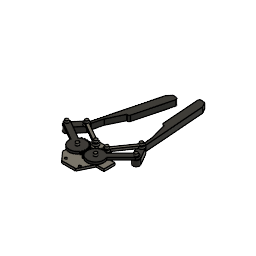
Record 11 (Autodesk Fusion 360 design; units mm, degrees)
part number: 2025-10-11-10-03-09-255
part number: 2025-10-12-12-27-50-455
part number: 2025-10-12-12-41-17-092
part number: 2025-10-12-12-45-11-913
part number: 2025-10-12-13-17-20-818
part number: 2025-10-12-13-49-26-949
Autodesk Fusion 360 part; units mm, degrees
sketch "Sketch2" plane through (0, 0, 0) normal (0, 1, 0) x (1, 0, 0)
  line L0 (0, 0) -> (14.2, 0)
  line L1 (14.2, 0) -> (14.2, 20)
  line L2 (0, 0) -> (-12.1733, -24.993)
  line L3 (-12.1733, -24.993) -> (-37.1733, -24.993)
  line L4 (-37.1733, -24.993) -> (-51.09, -9.7775)
  line L5 (-51.09, -9.7775) -> (-51.09, 20.2225)
  line L6 (-51.09, 20.2225) -> (-31.8645, 38.417)
  line L7 (-31.8645, 38.417) -> (-11.8645, 38.417)
  line L8 (-11.8645, 38.417) -> (7.148, 20)
  line L9 (7.148, 20) -> (14.2, 20)
  dimension "d11" = 14.2
  dimension "d12" = 20
  dimension "d13" = 27.8
  dimension "d14" = 25
  dimension "d15" = 20.62
  dimension "d16" = 30
  dimension "d17" = 26.47
  dimension "d18" = 20
  dimension "d20" = 26.47
  dimension "d21" = 63.41
  dimension "d22" = 65.29
  constraint coincident L0.start L2.start
  constraint horizontal L0
  constraint perpendicular L0 L1
  constraint perpendicular L1 L3
  constraint vertical L5
  constraint horizontal L7
  constraint perpendicular L1 L9
  measures "d11" distance of L0.start L0.end
  measures "d12" distance of L0.end L1.end
  measures "d13" distance of L0.start L2.end
  measures "d14" distance of L2.end L3.end
  measures "d15" distance of L3.end L4.end
  measures "d16" distance of L4.end L5.end
  measures "d17" distance of L5.end L6.end
  measures "d18" distance of L6.end L7.end
  measures "d20" distance of L7.end L8.end
  measures "d21" distance of L3 L7
  measures "d22" distance of L1 L5
extrude "Extrude1" add sketch "Sketch2" along normal blind 4 makes body 1
sketch "Sketch3" plane through (0, 4, 0) normal (0, 1, 0) x (-1, 0, 0)
  line L0 (0, 0) -> (-14.2, 0)
  line L1 (-14.2, 0) -> (-14.2, -20)
  line L2 (-14.2, -20) -> (-7.148, -20)
  line L3 (-7.148, -20) -> (11.8645, -38.417)
  line L4 (11.8645, -38.417) -> (31.8645, -38.417)
  line L5 (31.8645, -38.417) -> (51.09, -20.2225)
  line L6 (51.09, -20.2225) -> (51.09, 9.7775)
  line L7 (51.09, 9.7775) -> (37.1733, 24.993)
  line L8 (37.1733, 24.993) -> (12.1733, 24.993)
  line L9 (12.1733, 24.993) -> (0, 0)
  circle A0 centre (31.8645, -31.417) radius 3
  circle A1 centre (11.8645, -31.417) radius 3
  circle A2 centre (44, -10.2225) radius 3
  line L10 (15, -7) -> (0, -7)
  arc A3 (0, -7) -> (0, -13) centre (0, -10) ccw
  line L11 (0, -13) -> (15, -13)
  arc A4 (15, -13) -> (15, -7) centre (15, -10) ccw
  line L12 (15, -10) -> (0, -10) construction
  circle A5 centre (37.1733, 17.3853) radius 2
  circle A6 centre (12.1733, 17.3853) radius 2
  dimension "d25" = 6
  dimension "d26" = 6
  dimension "d27" = 7
  dimension "d28" = 7
  dimension "d29" = 6
  dimension "d30" = 10
  dimension "d31" = 7.09
  dimension "d32" = 6
  dimension "d33" = 14.2
  dimension "d34" = 10
  dimension "d35" = 4
  dimension "d36" = 4
  constraint tangent L10 A3
  constraint tangent A3 L11
  constraint parallel L10 L11
  constraint tangent L11 A4
  constraint tangent L10 A4
  constraint horizontal L12
  measures "d25" diameter of A0
  measures "d26" diameter of A1
  measures "d27" distance of L4.end A0.centre
  measures "d28" distance of L3.end A1.centre
  measures "d29" diameter of A2
  measures "d30" vertical distance of L5.end A2.centre
  measures "d31" distance of L6 A2.centre
  measures "d32" diameter of A3
  measures "d33" distance of L1 A3.centre
  measures "d34" distance of L2 A3.centre
  measures "d35" diameter of A5
  measures "d36" diameter of A6
extrude "Extrude2" cut sketch "Sketch3" against normal blind 33 contours A0 | A1 | A2 | L10 A3 L11 A4 | A5 | A6 bodies 1
sketch "Sketch1" plane through (0, 0, 0) normal (0, 1, 0) x (1, 0, 0) in component "part2"
  circle A0 centre (20.4961, 19.7492) radius 3
  line L0 (20.4961, 19.7492) -> (20.4961, -25.2508)
  circle A1 centre (20.4961, -25.2508) radius 3
  line L1 (17.9959, 15.4192) -> (17.9959, -20.9208)
  line L2 (22.9963, 15.4192) -> (22.9963, -20.9208)
  arc A2 (22.9963, 15.4192) -> (17.9959, 15.4192) centre (20.4961, 19.7492) ccw
  arc A3 (17.9959, -20.9208) -> (22.9963, -20.9208) centre (20.4961, -25.2508) ccw
  dimension "d39" = 10
  dimension "d40" = 6
  dimension "d41" = 45
  dimension "d42" = 10
  dimension "d43" = 6
  dimension "d44" = 36.34
  constraint concentric A0 A2
  constraint coincident A0.centre L0.start
  constraint vertical L0
  constraint coincident L0.end A1.centre
  constraint concentric A1 A3
  constraint vertical L1
  constraint symmetric L0 L1.start L2.start
  constraint symmetric L0 L1.end L2.end
  measures "d39" diameter of A2
  measures "d40" diameter of A0
  measures "d41" distance of A0.centre L0.end
  measures "d42" diameter of A3
  measures "d43" diameter of A1
  measures "d44" distance of L1.start L1.end
extrude "Extrude1'" add sketch "Sketch1" along normal blind 4 separate body makes body 2 in component "part2"
sketch "Sketch1 (2)" plane through (0, 0, 0) normal (0, 1, 0) x (1, 0, 0) in component "part 3"
  circle A0 centre (32, 23) radius 3
  dimension "d47" = 6
  measures "d47" diameter of A0
extrude "Extrude1''" add sketch "Sketch1 (2)" along normal blind 18 separate body makes body 3 in component "part 3"
sketch "Sketch1 (3)" plane through (0, 0, 0) normal (0, 1, 0) x (1, 0, 0) in component "part 4"
  circle A0 centre (-75.4732, 20.9598) radius 3
  line L0 (-75.4732, 20.9598) -> (-75.4732, -31.0102)
  circle A1 centre (-75.4732, -31.0102) radius 3
  line L1 (-80.3495, -29.9048) -> (-80.3495, 6.7746)
  line L2 (-70.597, -29.9048) -> (-70.597, 6.7746)
  arc A2 (-80.3495, -29.9048) -> (-70.597, -29.9048) centre (-75.4732, -31.0102) ccw
  line L3 (-75.4732, 20.9598) -> (-75.4732, 40)
  line L4 (-76.5054, 35.9243) -> (-76.5054, 37.4643)
  line L5 (-76.5054, 37.4643) -> (-76.5054, 35.9243)
  line L6 (-76.5054, 37.4643) -> (-75.9732, 37.9343)
  line L7 (-75.9732, 37.9343) -> (-75.4732, 37.9343)
  line L8 (-74.4411, 37.4643) -> (-74.4411, 35.9243)
  line L9 (-74.4411, 37.4643) -> (-74.9732, 37.9343)
  line L10 (-74.9732, 37.9343) -> (-75.4732, 37.9343)
  line L11 (-80.2193, 35.1892) -> (-80.6049, 36.6801)
  line L12 (-80.6049, 36.6801) -> (-80.2074, 37.2684)
  line L13 (-80.2074, 37.2684) -> (-79.7233, 37.3936)
  line L14 (-79.2392, 37.5188) -> (-79.7233, 37.3936)
  line L15 (-78.6063, 37.197) -> (-79.2392, 37.5188)
  line L16 (-78.6063, 37.197) -> (-78.2208, 35.706)
  line L17 (-83.6309, 33.5476) -> (-84.3775, 34.8945)
  line L18 (-84.3775, 34.8945) -> (-84.1399, 35.5636)
  line L19 (-84.1399, 35.5636) -> (-83.7026, 35.806)
  line L20 (-83.2653, 36.0484) -> (-83.7026, 35.806)
  line L21 (-82.572, 35.8953) -> (-83.2653, 36.0484)
  line L22 (-82.572, 35.8953) -> (-81.8254, 34.5484)
  line L23 (-86.5228, 31.1042) -> (-87.5829, 32.2212)
  line L24 (-87.5829, 32.2212) -> (-87.5204, 32.9285)
  line L25 (-87.5204, 32.9285) -> (-87.1577, 33.2726)
  line L26 (-86.795, 33.6168) -> (-87.1577, 33.2726)
  line L27 (-86.0854, 33.6422) -> (-86.795, 33.6168)
  line L28 (-86.0854, 33.6422) -> (-85.0254, 32.5251)
  line L29 (-88.7108, 28.0144) -> (-90.0168, 28.8305)
  line L30 (-90.0168, 28.8305) -> (-90.1333, 29.5309)
  line L31 (-90.1333, 29.5309) -> (-89.8684, 29.9549)
  line L32 (-89.6034, 30.3789) -> (-89.8684, 29.9549)
  line L33 (-88.9228, 30.5812) -> (-89.6034, 30.3789)
  line L34 (-88.9228, 30.5812) -> (-87.6168, 29.7651)
  line L35 (-90.0555, 24.4753) -> (-91.5242, 24.9384)
  line L36 (-91.5242, 24.9384) -> (-91.8124, 25.5873)
  line L37 (-91.8124, 25.5873) -> (-91.6621, 26.0641)
  line L38 (-91.5117, 26.541) -> (-91.6621, 26.0641)
  line L39 (-90.9034, 26.9072) -> (-91.5117, 26.541)
  line L40 (-90.9034, 26.9072) -> (-89.4347, 26.4441)
  line L41 (-90.4712, 20.7122) -> (-92.0091, 20.7928)
  line L42 (-92.0091, 20.7928) -> (-92.4506, 21.3489)
  line L43 (-92.4506, 21.3489) -> (-92.4244, 21.8482)
  line L44 (-92.3983, 22.3475) -> (-92.4244, 21.8482)
  line L45 (-91.901, 22.8543) -> (-92.3983, 22.3475)
  line L46 (-91.901, 22.8543) -> (-90.3632, 22.7738)
  line L47 (-89.9315, 16.9649) -> (-91.4406, 16.6579)
  line L48 (-91.4406, 16.6579) -> (-92.0072, 17.0857)
  line L49 (-92.0072, 17.0857) -> (-92.1069, 17.5757)
  line L50 (-92.2066, 18.0656) -> (-92.1069, 17.5757)
  line L51 (-91.8521, 18.6808) -> (-92.2066, 18.0656)
  line L52 (-91.8521, 18.6808) -> (-90.3431, 18.9878)
  line L53 (-88.4707, 13.4721) -> (-89.8549, 12.797)
  line L54 (-89.8549, 12.797) -> (-90.5106, 13.0693)
  line L55 (-90.5106, 13.0693) -> (-90.7298, 13.5187)
  line L56 (-90.949, 13.9681) -> (-90.7298, 13.5187)
  line L57 (-90.7598, 14.6525) -> (-90.949, 13.9681)
  line L58 (-90.7598, 14.6525) -> (-89.3757, 15.3275)
  line L59 (-86.182, 10.4563) -> (-87.353, 9.4562)
  line L60 (-87.353, 9.4562) -> (-88.056, 9.5556)
  line L61 (-88.056, 9.5556) -> (-88.3807, 9.9358)
  line L62 (-88.7054, 10.316) -> (-88.3807, 9.9358)
  line L63 (-88.6937, 11.0259) -> (-88.7054, 10.316)
  line L64 (-88.6937, 11.0259) -> (-87.5226, 12.0261)
  line L65 (-83.211, 8.1096) -> (-84.0943, 6.8481)
  line L66 (-84.0943, 6.8481) -> (-84.7998, 6.7684)
  line L67 (-84.7998, 6.7684) -> (-85.2094, 7.0552)
  line L68 (-85.619, 7.342) -> (-85.2094, 7.0552)
  line L69 (-85.7853, 8.0322) -> (-85.619, 7.342)
  line L70 (-85.7853, 8.0322) -> (-84.902, 9.2937)
  arc A3 (-70.597, 6.7746) -> (-74.4411, 35.9243) centre (-75.4732, 20.9598) ccw
  arc A4 (-76.5054, 35.9243) -> (-78.2208, 35.706) centre (-75.4732, 20.9598) ccw
  arc A5 (-80.2193, 35.1892) -> (-81.8254, 34.5484) centre (-75.4732, 20.9598) ccw
  arc A6 (-83.6309, 33.5476) -> (-85.0254, 32.5251) centre (-75.4732, 20.9598) ccw
  arc A7 (-86.5228, 31.1042) -> (-87.6168, 29.7651) centre (-75.4732, 20.9598) ccw
  arc A8 (-88.7108, 28.0144) -> (-89.4347, 26.4441) centre (-75.4732, 20.9598) ccw
  arc A9 (-90.0555, 24.4753) -> (-90.3632, 22.7738) centre (-75.4732, 20.9598) ccw
  arc A10 (-90.4712, 20.7122) -> (-90.3431, 18.9878) centre (-75.4732, 20.9598) ccw
  arc A11 (-89.9315, 16.9649) -> (-89.3757, 15.3275) centre (-75.4732, 20.9598) ccw
  arc A12 (-88.4707, 13.4721) -> (-87.5226, 12.0261) centre (-75.4732, 20.9598) ccw
  arc A13 (-86.182, 10.4563) -> (-84.902, 9.2937) centre (-75.4732, 20.9598) ccw
  arc A14 (-83.211, 8.1096) -> (-80.3495, 6.7746) centre (-75.4732, 20.9598) ccw
  dimension "d50" = 30
  dimension "d51" = 6
  dimension "d52" = 10
  dimension "d53" = 6
  dimension "d54" = 51.97
  dimension "d55" = 1.54
  dimension "d56" = 0.47
  dimension "d57" = 0.5
  dimension "d58" = 0.71
  dimension "d60" = 145
  constraint concentric A0 A3
  constraint coincident A0.centre L0.start
  constraint vertical L0
  constraint coincident L0.end A1.centre
  constraint concentric A1 A2
  constraint parallel L0 L1
  constraint symmetric L0 L1.start L2.start
  constraint symmetric L0 L1.end L2.end
  constraint parallel L0 L3
  constraint vertical L4
  constraint coincident L4.start A3
  constraint coincident L3 L7.end
  constraint perpendicular L3 L7
  constraint symmetric L3 L4.start L8.end
  constraint symmetric L3 L4.end L8.start
  constraint symmetric L3 L6.end L9.end
  constraint symmetric L3 L7.end L10.end
  constraint concentric A3 A4
  constraint concentric A4 A5
  constraint concentric A5 A6
  constraint concentric A6 A7
  constraint concentric A7 A8
  constraint concentric A8 A9
  constraint concentric A9 A10
  constraint concentric A10 A11
  constraint concentric A11 A12
  constraint concentric A12 A13
  constraint concentric A13 A14
  measures "d50" diameter of A3
  measures "d51" diameter of A0
  measures "d52" diameter of A2
  measures "d53" diameter of A1
  measures "d54" distance of A0.centre L0.end
  measures "d55" distance of L4.start L4.end
  measures "d56" vertical distance of L4.end L6.end
  measures "d57" distance of L6.end L7.end
  measures "d58" distance of L4.end L6.end
extrude "Extrude1'''" add sketch "Sketch1 (3)" along normal blind 4 separate body makes body 4 in component "part 4"
sketch "Sketch1 (4)" plane through (0, 0, 0) normal (0, 1, 0) x (1, 0, 0) in component "part 5"
  line L0 (79.2313, -48.7678) -> (79.2313, -23.7678)
  arc A0 (79.2313, -23.7678) -> (67.2313, -23.7678) centre (73.2313, -23.7678) ccw
  line L1 (67.2313, -23.7678) -> (67.2313, -48.7678)
  arc A1 (67.2313, -48.7678) -> (79.2313, -48.7678) centre (73.2313, -48.7678) ccw
  line L2 (73.2313, -48.7678) -> (73.2313, -23.7678) construction
  line L3 (69.067, -19.4483) -> (20.2413, 82.4588)
  line L4 (20.2413, 82.4588) -> (20.2413, 92.3588)
  line L5 (26.0982, 96.1925) -> (20.2413, 92.3588)
  line L6 (30.4467, 94.9786) -> (59.6439, 34.0394)
  arc A2 (30.4467, 94.9786) -> (26.0982, 96.1925) centre (27.7412, 93.6824) ccw
  line L7 (77.8305, -27.1163) -> (64.8679, -0.0613)
  line L8 (58.2346, 30.0376) -> (57.3328, 29.6055)
  line L9 (57.3328, 29.6055) -> (64.8679, -0.0613)
  arc A3 (58.2346, 30.0376) -> (59.6439, 34.0394) centre (56.9384, 32.7431) ccw
  point P0 (28.9658, 98.0695)
  point P1 (60.9401, 31.3339)
  dimension "d63" = 25
  dimension "d64" = 12
  dimension "d65" = 113
  dimension "d66" = 154.4
  dimension "d67" = 58.99
  dimension "d68" = 9.9
  dimension "d69" = 74
  dimension "d70" = 3
  dimension "d71" = 7
  dimension "d72" = 30
  dimension "d73" = 4.59
  dimension "d74" = 3
  dimension "d75" = 1
  constraint tangent L0 A0
  constraint tangent A0 L1
  constraint parallel L0 L1
  constraint tangent L1 A1
  constraint tangent L0 A1
  constraint vertical L2
  constraint coincident A0 L3.start
  constraint vertical L4
  constraint parallel L3 L6
  constraint coincident P0 L5
  constraint coincident P0 L6
  constraint tangent L5 A2
  constraint tangent L6 A2
  constraint parallel L3 L7
  constraint perpendicular L6 L8
  constraint coincident P1 L6
  constraint coincident P1 L8
  constraint tangent L6 A3
  constraint tangent L8 A3
  measures "d63" distance of A1.centre A0.centre
  measures "d64" diameter of A0
  measures "d65" distance of L3.start L3.end
  measures "d66" angle of L1 L3
  measures "d67" distance of L0 L3.end
  measures "d68" distance of L3.end L4.end
  measures "d69" distance of P0 P1
  measures "d70" radius of A2
  measures "d71" distance of L4.end L5.start
  measures "d72" distance of L7.start L7.end
  measures "d73" distance of L3 L7
  measures "d74" radius of A3
  measures "d75" distance of L8.end L8.start
extrude "Extrude1''''" add sketch "Sketch1 (4)" along normal blind 10 separate body makes body 5 in component "part 5"
sketch "Sketch2 (2)" plane through (0, 10, 0) normal (0, 1, 0) x (-1, 0, 0) in component "part 5"
  line L0 (-57.3328, -29.6055) -> (-58.2346, -30.0376)
  arc A0 (-58.2346, -30.0376) -> (-59.6439, -34.0394) centre (-56.9384, -32.7431) ccw
  line L1 (-59.6439, -34.0394) -> (-30.4467, -94.9786)
  arc A1 (-30.4467, -94.9786) -> (-26.0982, -96.1925) centre (-27.7412, -93.6824) ccw
  line L2 (-26.0982, -96.1925) -> (-20.2413, -92.3588)
  line L3 (-20.2413, -92.3588) -> (-20.2413, -82.4588)
  line L4 (-20.2413, -82.4588) -> (-69.067, 19.4483)
  arc A2 (-69.067, 19.4483) -> (-67.2313, 23.7678) centre (-73.2313, 23.7678) ccw
  line L5 (-67.2313, 23.7678) -> (-67.2313, 48.7678)
  arc A3 (-67.2313, 48.7678) -> (-79.2313, 48.7678) centre (-73.2313, 48.7678) ccw
  line L6 (-79.2313, 48.7678) -> (-79.2313, 23.7678)
  arc A4 (-79.2313, 23.7678) -> (-73.3521, 17.7691) centre (-73.2313, 23.7678) ccw
  line L7 (-73.3521, 17.7691) -> (-64.8679, 0.0613)
  line L8 (-64.8679, 0.0613) -> (-57.3328, -29.6055)
  circle A5 centre (-73.2313, 48.7678) radius 3
  circle A6 centre (-73.2313, 23.7678) radius 3
  dimension "d78" = 6
  dimension "d79" = 6
  constraint concentric A3 A5
  constraint concentric A2 A6
  measures "d78" diameter of A5
  measures "d79" diameter of A6
extrude "Extrude2'" cut sketch "Sketch2 (2)" against normal blind 40 contours A5 | A6 bodies 5 in component "part 5"
component "part2" placed x (0.5, 0, -0.866025) y (0, 1, 0) z (0.866025, 0, 0.5) at (-63.9803, 4, -26.2923)
component "part 3" placed x (0.866025, 0, 0.5) y (0, 1, 0) z (-0.5, 0, 0.866025) at (-83.2128, -6, -6.3039)
component "part 4" placed x (-0.5, 0, 0.866025) y (0, 1, 0) z (-0.866025, 0, -0.5) at (-99.8884, 4, 44.6594)
component "part 5" placed x (0.766044, 0, 0.642788) y (0, 1, 0) z (-0.642788, 0, 0.766044) at (-113.7584, -6, -120.638)
component "Component" placed x (1, 0, 0) y (0, 1, 0) z (0, 0, 1) at (0, 0, 0)
component "part 3" placed x (0.866025, 0, 0.5) y (0, 1, 0) z (-0.5, 0, 0.866025) at (-128.2202, -6, -32.2889)
component "part 3" placed x (0.866025, 0, 0.5) y (0, 1, 0) z (-0.5, 0, 0.866025) at (-110.0485, -6, -49.9984)
component "part 3" placed x (0.866025, 0, 0.5) y (0, 1, 0) z (-0.5, 0, 0.866025) at (-71.0773, -6, -27.4984)
component "part 4" placed x (-0.5, 0, 0.866025) y (0, 1, 0) z (-0.866025, 0, -0.5) at (-99.8884, 4, 44.6594)
component "part 4" placed x (-0.5, 0, 0.866025) y (0, 1, 0) z (-0.866025, 0, -0.5) at (-99.8884, 4, 44.6594)
component "part 4" placed x (0.707107, 0, 0.707107) y (0, -1, 0) z (0.707107, 0, -0.707107) at (57.1885, 8, 28.5468)
component "part 5" placed x (0.766044, 0, 0.642788) y (0, 1, 0) z (-0.642788, 0, 0.766044) at (-113.7584, -6, -120.638)
component "part 5" placed x (-0.866025, 0, 0.5) y (0, -1, 0) z (0.5, 0, 0.866025) at (64.7846, 4, -125.5982)
component "part 3" placed x (0.707107, 0, 0.707107) y (0, 1, 0) z (-0.707107, 0, 0.707107) at (-13.1425, -6, -53.1123)
component "part2" placed x (0.819152, 0, 0.573576) y (0, 1, 0) z (-0.573576, 0, 0.819152) at (-14.1707, 4, -63.8573)
component "part 3" placed x (0.819152, 0, 0.573576) y (0, 1, 0) z (-0.573576, 0, 0.819152) at (-51.2696, -6, -30.9309)
component "part 3" placed x (0.707107, 0, 0.707107) y (0, 1, 0) z (-0.707107, 0, 0.707107) at (-49.8909, -6, -16.364)
component "part 3" placed x (0.819152, 0, 0.573576) y (0, 1, 0) z (-0.573576, 0, 0.819152) at (-25.4587, -6, -67.7928)
equation "d54 = 71.97 mm - 15 mm - 5 mm"
